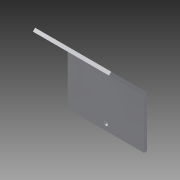
# Autodesk Inventor part: camera mount
Saved by Autodesk Inventor 2015 SP1 (Build 190203100, 203)
## iProperties
Created: 2015-01-18
Part Number: camera mount
Material: Generic
Document SubType Name: Modeling
Designer: Jarod
Density: 1 g/cm^3
Appearance: Default
Author: Jarod
Autodesk Inventor part; units mm, degrees
ref_plane "YZ Plane" through (0, 0, 0) normal (1, 0, 0) x (0, 1, 0)
ref_plane "XZ Plane" through (0, 0, 0) normal (0, 1, 0) x (-1, 0, 0)
ref_plane "XY Plane" through (0, 0, 0) normal (0, 0, 1) x (1, 0, 0)
sketch "Sketch1" plane through (0, 0, 0) normal (1, 0, 0) x (0, 1, 0)
  line L0 (0, 0) -> (-50.8, 0)
  line L1 (-50.8, 0) -> (-50.8, 3.175)
  line L2 (-50.8, 3.175) -> (0, 3.175)
  line L3 (0, 3.175) -> (0, 0)
  line L4 (0, 0) -> (35.921, 35.921)
  line L5 (35.921, 35.921) -> (33.676, 38.1661)
  line L6 (33.676, 38.1661) -> (-2.2451, 2.2451)
  line L7 (-2.2451, 2.2451) -> (0, 0)
  line L8 (0, 0) -> (50.8, 0) construction
  dimension "d0" = 50.8
  dimension "d1" = 3.175
  dimension "d2" = 50.8
  dimension "d3" = 45
  dimension "d4" = 3.175
  constraints: 18 end point, 4 parallel, 2 horizontal, 2 perpendicular, 1 equal length
  measures "d0" distance of L1.end L2.end
  measures "d1" distance of L0.end L1.end
  measures "d2" distance of L0.start L4.end
  measures "d3" angle of L8 L4
  measures "d4" distance of L5.end L4.end
extrude "Extrusion1" add sketch "Sketch1" along normal blind 76.2
sketch "Sketch2" plane through (76.2, 35.921, 35.921) normal (0, 0.7071068, -0.7071068) x (-1, 0, 0)
  line L0 (76.2, -50.8) -> (76.2, 0) projected
  line L1 (76.2, 0) -> (0, 0) projected
  line L2 (0, -50.8) -> (0, 0) projected
  line L3 (76.2, -50.8) -> (0, -50.8) projected
  point P0 (12.7, -12.7)
  point P1 (63.5, -12.7)
  dimension "d7" = 38.1
  dimension "d8" = 38.1
  dimension "d9" = 12.7
  dimension "d10" = 12.7
  measures "d7" distance from line of point (63.5, -12.7) L3
  measures "d8" distance from line of L3 point (12.7, -12.7)
  measures "d9" distance from line of L2 point (12.7, -12.7)
  measures "d10" distance from line of L0 point (63.5, -12.7)
hole "Hole1" at (63.5, 26.9408, 26.9408) at (12.7, 26.9408, 26.9408) direction (0, -0.7071068, 0.7071068) diameter 6.35 end through all
sketch "Sketch3" plane through (0, -50.8, 0) normal (0, 0, -1) x (-1, 0, 0)
  line L0 (0, 0) -> (0, 50.8) projected
  line L1 (0, 50.8) -> (-76.2, 50.8) projected
  line L2 (-76.2, 0) -> (-76.2, 50.8) projected
  line L3 (0, 0) -> (-76.2, 0) projected
  point P0 (-38.1, 6.35)
  dimension "d18" = 6.35
  dimension "d19" = 38.1
  measures "d18" distance from line of L3 point (-38.1, 6.35)
  measures "d19" distance from line of L0 point (-38.1, 6.35)
hole "Hole2" at (38.1, -44.45, 0) direction (0, 0, 1) diameter 3.9688 end through all
body "Solid1"
